Autodesk Inventor part; units mm, degrees
(part 3 of 5)
  spline S419 degree 2 poles (-346.7745, 60.714) (-347.3687, 60.714) (-348.0307, 61.3279) (-348.0307, 61.8712) knots 0 0 0 1 2 2 2
  spline S420 degree 2 poles (-348.0307, 61.8712) (-348.0307, 62.2163) (-347.7195, 62.7284) (-347.1452, 63) (-346.7717, 63) knots 0 0 0 1 2 3 3 3
  spline S421 degree 2 poles (-346.7717, 63) (-346.3841, 63) (-345.8154, 62.7143) (-345.5126, 62.2078) (-345.5126, 61.8966) knots 0 0 0 1 2 3 3 3
  spline S422 degree 2 poles (-346.4322, 61.891) (-346.4322, 62.3352) (-346.7717, 62.3352) knots 0 0 0 1 1 1
  spline S423 degree 2 poles (-346.7717, 62.3352) (-347.1112, 62.3352) (-347.1112, 61.8712) knots 0 0 0 1 1 1
  spline S424 degree 2 poles (-347.1112, 61.8712) (-347.1112, 61.3789) (-346.766, 61.3789) knots 0 0 0 1 1 1
  spline S425 degree 2 poles (-346.766, 61.3789) (-346.4322, 61.3789) (-346.4322, 61.891) knots 0 0 0 1 1 1
  spline S426 degree 2 poles (-398.07, 55.8694) (-398.07, 55.7053) (-398.2397, 55.4139) (-398.5311, 55.247) (-398.6924, 55.247) knots 0 0 0 1 2 3 3 3
  spline S427 degree 2 poles (-398.6924, 55.247) (-398.9442, 55.247) (-399.3064, 55.6091) (-399.3064, 55.8694) knots 0 0 0 1 2 2 2
  spline S428 degree 2 poles (-399.3064, 55.8694) (-399.3064, 56.1212) (-398.9499, 56.4834) (-398.6924, 56.4834) knots 0 0 0 1 2 2 2
  spline S429 degree 2 poles (-398.6924, 56.4834) (-398.4293, 56.4834) (-398.07, 56.1156) (-398.07, 55.8694) knots 0 0 0 1 2 2 2
  spline S430 degree 2 poles (-387.3157, 56.3957) (-387.3157, 55.9317) (-387.7062, 55.2187) (-388.4277, 54.8311) (-388.9002, 54.8311) knots 0 0 0 1 2 3 3 3
  line L463 (-388.9002, 54.8311) -> (-390.1932, 54.8311)
  line L464 (-390.1932, 54.8311) -> (-390.1932, 57.8811)
  line L465 (-390.1932, 57.8811) -> (-388.9285, 57.8811)
  spline S431 degree 2 poles (-388.9285, 57.8811) (-387.3157, 57.8811) (-387.3157, 56.3957) knots 0 0 0 1 1 1
  spline S432 degree 2 poles (-388.2919, 56.3872) (-388.2919, 56.6079) (-388.4729, 56.9672) (-388.8096, 57.1624) (-389.036, 57.1624) knots 0 0 0 1 2 3 3 3
  line L466 (-389.036, 57.1624) -> (-389.2736, 57.1624)
  line L467 (-389.2736, 57.1624) -> (-389.2736, 55.5497)
  line L468 (-389.2736, 55.5497) -> (-389.0162, 55.5497)
  spline S433 degree 2 poles (-389.0162, 55.5497) (-388.6851, 55.5497) (-388.2919, 56.0024) (-388.2919, 56.3872) knots 0 0 0 1 2 2 2
  spline S434 degree 2 poles (-386.1868, 55.6629) (-386.1642, 55.5214) (-385.8869, 55.363) (-385.6606, 55.363) knots 0 0 0 1 2 2 2
  spline S435 degree 2 poles (-385.6606, 55.363) (-385.3437, 55.363) (-385.0608, 55.4846) knots 0 0 0 1 1 1
  line L469 (-385.0608, 55.4846) -> (-385.0608, 54.9103)
  spline S436 degree 2 poles (-385.0608, 54.9103) (-385.389, 54.7773) (-385.8615, 54.7773) knots 0 0 0 1 1 1
  spline S437 degree 2 poles (-385.8615, 54.7773) (-386.4302, 54.7773) (-387.0639, 55.3601) (-387.0639, 55.8722) knots 0 0 0 1 2 2 2
  spline S438 degree 2 poles (-387.0639, 55.8722) (-387.0639, 56.2231) (-386.7867, 56.7578) (-386.2406, 57.0634) (-385.9096, 57.0634) knots 0 0 0 1 2 3 3 3
  spline S439 degree 2 poles (-385.9096, 57.0634) (-385.5729, 57.0634) (-385.0919, 56.8003) (-384.8429, 56.3221) (-384.8429, 56.0024) knots 0 0 0 1 2 3 3 3
  line L470 (-384.8429, 56.0024) -> (-384.8429, 55.6629)
  line L471 (-384.8429, 55.6629) -> (-386.1868, 55.6629)
  spline S440 degree 2 poles (-385.6436, 56.1382) (-385.6436, 56.5145) (-385.9124, 56.5145) knots 0 0 0 1 1 1
  spline S441 degree 2 poles (-385.9124, 56.5145) (-386.0256, 56.5145) (-386.1784, 56.308) (-386.1925, 56.1382) knots 0 0 0 1 2 2 2
  line L472 (-386.1925, 56.1382) -> (-385.6436, 56.1382)
  line L473 (-384.5289, 54.8311) -> (-384.5289, 58.0565)
  line L474 (-384.5289, 58.0565) -> (-383.6235, 58.0565)
  line L475 (-383.6235, 58.0565) -> (-383.6235, 54.8311)
  line L476 (-383.6235, 54.8311) -> (-384.5289, 54.8311)
  spline S442 degree 2 poles (-379.3993, 56.8766) (-379.3993, 56.5626) (-379.7162, 56.0788) (-380.3047, 55.8128) (-380.6952, 55.8128) knots 0 0 0 1 2 3 3 3
  line L477 (-380.6952, 55.8128) -> (-380.9753, 55.8128)
  line L478 (-380.9753, 55.8128) -> (-380.9753, 54.8311)
  line L479 (-380.9753, 54.8311) -> (-381.8948, 54.8311)
  line L480 (-381.8948, 54.8311) -> (-381.8948, 57.8811)
  line L481 (-381.8948, 57.8811) -> (-380.6414, 57.8811)
  spline S443 degree 2 poles (-380.6414, 57.8811) (-379.9963, 57.8811) (-379.3993, 57.3916) (-379.3993, 56.8766) knots 0 0 0 1 2 2 2
  spline S444 degree 2 poles (-380.3726, 56.8427) (-380.3726, 57.0294) (-380.5905, 57.2218) (-380.7998, 57.2218) knots 0 0 0 1 2 2 2
  line L482 (-380.7998, 57.2218) -> (-380.9753, 57.2218)
  line L483 (-380.9753, 57.2218) -> (-380.9753, 56.4692)
  line L484 (-380.9753, 56.4692) -> (-380.7687, 56.4692)
  spline S445 degree 2 poles (-380.7687, 56.4692) (-380.3726, 56.4692) (-380.3726, 56.8427) knots 0 0 0 1 1 1
  line L485 (-377.9111, 54.8311) -> (-377.9111, 55.1621)
  line L486 (-377.9111, 55.1621) -> (-377.9196, 55.1621)
  spline S446 degree 2 poles (-377.9196, 55.1621) (-378.1375, 54.7773) (-378.5845, 54.7773) knots 0 0 0 1 1 1
  spline S447 degree 2 poles (-378.5845, 54.7773) (-378.8929, 54.7773) (-379.2409, 55.1423) (-379.2409, 55.4507) knots 0 0 0 1 2 2 2
  spline S448 degree 2 poles (-379.2409, 55.4507) (-379.2409, 56.0929) (-378.4515, 56.1948) knots 0 0 0 1 1 1
  line L487 (-378.4515, 56.1948) -> (-377.9111, 56.2655)
  spline S449 degree 2 poles (-377.9111, 56.2655) (-377.9111, 56.373) (-378.1035, 56.5088) (-378.2648, 56.5088) knots 0 0 0 1 2 2 2
  spline S450 degree 2 poles (-378.2648, 56.5088) (-378.6298, 56.5088) (-379.0372, 56.2995) knots 0 0 0 1 1 1
  line L488 (-379.0372, 56.2995) -> (-379.0372, 56.888)
  spline S451 degree 2 poles (-379.0372, 56.888) (-378.8618, 56.9644) (-378.327, 57.0634) (-378.1375, 57.0634) knots 0 0 0 1 2 2 2
  spline S452 degree 2 poles (-378.1375, 57.0634) (-377.5829, 57.0634) (-377.0821, 56.5881) (-377.0821, 56.0335) knots 0 0 0 1 2 2 2
  line L489 (-377.0821, 56.0335) -> (-377.0821, 54.8311)
  line L490 (-377.0821, 54.8311) -> (-377.9111, 54.8311)
  spline S453 degree 2 poles (-378.4487, 55.5723) (-378.4487, 55.4846) (-378.3355, 55.3686) (-378.2308, 55.3686) knots 0 0 0 1 2 2 2
  spline S454 degree 2 poles (-378.2308, 55.3686) (-378.0894, 55.3686) (-377.9111, 55.5808) (-377.9111, 55.7478) knots 0 0 0 1 2 2 2
  line L491 (-377.9111, 55.7478) -> (-377.9111, 55.8298)
  line L492 (-377.9111, 55.8298) -> (-378.2195, 55.7874)
  spline S455 degree 2 poles (-378.2195, 55.7874) (-378.4487, 55.7478) (-378.4487, 55.5723) knots 0 0 0 1 1 1
  spline S456 degree 2 poles (-374.2189, 55.9854) (-374.2189, 55.6289) (-374.4622, 55.08) (-374.9035, 54.7773) (-375.1808, 54.7773) knots 0 0 0 1 2 3 3 3
  spline S457 degree 2 poles (-375.1808, 54.7773) (-375.5628, 54.7773) (-375.7608, 55.0574) knots 0 0 0 1 1 1
  line L493 (-375.7608, 55.0574) -> (-375.7693, 55.0574)
  line L494 (-375.7693, 55.0574) -> (-375.7693, 53.8295)
  line L495 (-375.7693, 53.8295) -> (-376.6747, 53.8295)
  line L496 (-376.6747, 53.8295) -> (-376.6747, 57.0096)
  line L497 (-376.6747, 57.0096) -> (-375.7693, 57.0096)
  line L498 (-375.7693, 57.0096) -> (-375.7693, 56.7125)
  line L499 (-375.7693, 56.7125) -> (-375.7608, 56.7125)
  spline S458 degree 2 poles (-375.7608, 56.7125) (-375.6533, 56.8766) (-375.3081, 57.0634) (-375.0875, 57.0634) knots 0 0 0 1 2 2 2
  spline S459 degree 2 poles (-375.0875, 57.0634) (-374.6687, 57.0634) (-374.2189, 56.5004) (-374.2189, 55.9854) knots 0 0 0 1 2 2 2
  spline S460 degree 2 poles (-375.1384, 55.96) (-375.1384, 56.1637) (-375.2968, 56.3985) (-375.4638, 56.3985) knots 0 0 0 1 2 2 2
  spline S461 degree 2 poles (-375.4638, 56.3985) (-375.608, 56.3985) (-375.7863, 56.1523) (-375.7863, 55.9373) knots 0 0 0 1 2 2 2
  line L500 (-375.7863, 55.9373) -> (-375.7863, 55.8949)
  spline S462 degree 2 poles (-375.7863, 55.8949) (-375.7863, 55.6883) (-375.6335, 55.4422) (-375.4807, 55.4422) knots 0 0 0 1 2 2 2
  spline S463 degree 2 poles (-375.4807, 55.4422) (-375.3166, 55.4422) (-375.1384, 55.711) (-375.1384, 55.96) knots 0 0 0 1 2 2 2
  line L501 (-372.6684, 54.8311) -> (-372.6684, 55.1621)
  line L502 (-372.6684, 55.1621) -> (-372.6769, 55.1621)
  spline S464 degree 2 poles (-372.6769, 55.1621) (-372.8947, 54.7773) (-373.3418, 54.7773) knots 0 0 0 1 1 1
  spline S465 degree 2 poles (-373.3418, 54.7773) (-373.6502, 54.7773) (-373.9982, 55.1423) (-373.9982, 55.4507) knots 0 0 0 1 2 2 2
  spline S466 degree 2 poles (-373.9982, 55.4507) (-373.9982, 56.0929) (-373.2088, 56.1948) knots 0 0 0 1 1 1
  line L503 (-373.2088, 56.1948) -> (-372.6684, 56.2655)
  spline S467 degree 2 poles (-372.6684, 56.2655) (-372.6684, 56.373) (-372.8608, 56.5088) (-373.0221, 56.5088) knots 0 0 0 1 2 2 2
  spline S468 degree 2 poles (-373.0221, 56.5088) (-373.387, 56.5088) (-373.7945, 56.2995) knots 0 0 0 1 1 1
  line L504 (-373.7945, 56.2995) -> (-373.7945, 56.888)
  spline S469 degree 2 poles (-373.7945, 56.888) (-373.619, 56.9644) (-373.0843, 57.0634) (-372.8947, 57.0634) knots 0 0 0 1 2 2 2
  spline S470 degree 2 poles (-372.8947, 57.0634) (-372.3402, 57.0634) (-371.8394, 56.5881) (-371.8394, 56.0335) knots 0 0 0 1 2 2 2
  line L505 (-371.8394, 56.0335) -> (-371.8394, 54.8311)
  line L506 (-371.8394, 54.8311) -> (-372.6684, 54.8311)
  line L507 (-373.0277, 57.3548) -> (-373.786, 58.0367)
  line L508 (-373.786, 58.0367) -> (-373.0249, 58.0367)
  line L509 (-373.0249, 58.0367) -> (-372.3883, 57.3548)
  line L510 (-372.3883, 57.3548) -> (-373.0277, 57.3548)
  spline S471 degree 2 poles (-373.206, 55.5723) (-373.206, 55.4846) (-373.0928, 55.3686) (-372.9881, 55.3686) knots 0 0 0 1 2 2 2
  spline S472 degree 2 poles (-372.9881, 55.3686) (-372.8466, 55.3686) (-372.6684, 55.5808) (-372.6684, 55.7478) knots 0 0 0 1 2 2 2
  line L511 (-372.6684, 55.7478) -> (-372.6684, 55.8298)
  line L512 (-372.6684, 55.8298) -> (-372.9768, 55.7874)
  spline S473 degree 2 poles (-372.9768, 55.7874) (-373.206, 55.7478) (-373.206, 55.5723) knots 0 0 0 1 1 1
  line L513 (-368.0085, 54.8311) -> (-369.0836, 56.3023)
  spline S474 degree 2 poles (-369.0836, 56.3023) (-369.211, 56.4749) (-369.293, 56.6164) knots 0 0 0 1 1 1
  line L514 (-369.293, 56.6164) -> (-369.3015, 56.6164)
  spline S475 degree 2 poles (-369.3015, 56.6164) (-369.2874, 56.39) (-369.2874, 56.1099) knots 0 0 0 1 1 1
  line L515 (-369.2874, 56.1099) -> (-369.2874, 54.8311)
  line L516 (-369.2874, 54.8311) -> (-370.139, 54.8311)
  line L517 (-370.139, 54.8311) -> (-370.139, 57.8811)
  line L518 (-370.139, 57.8811) -> (-369.2704, 57.8811)
  line L519 (-369.2704, 57.8811) -> (-368.2405, 56.4805)
  spline S476 degree 2 poles (-368.2405, 56.4805) (-368.2207, 56.4523) (-368.1641, 56.3759) (-368.1104, 56.2966) (-368.0623, 56.2202) (-368.0481, 56.1891) knots 0 0 0 1 2 3 4 4 4
  line L520 (-368.0481, 56.1891) -> (-368.0396, 56.1891)
  spline S477 degree 2 poles (-368.0396, 56.1891) (-368.0538, 56.2825) (-368.0538, 56.5117) knots 0 0 0 1 1 1
  line L521 (-368.0538, 56.5117) -> (-368.0538, 57.8811)
  line L522 (-368.0538, 57.8811) -> (-367.2022, 57.8811)
  line L523 (-367.2022, 57.8811) -> (-367.2022, 54.8311)
  line L524 (-367.2022, 54.8311) -> (-368.0085, 54.8311)
  line L525 (-366.6844, 54.8311) -> (-366.6844, 57.0096)
  line L526 (-366.6844, 57.0096) -> (-365.779, 57.0096)
  line L527 (-365.779, 57.0096) -> (-365.779, 54.8311)
  line L528 (-365.779, 54.8311) -> (-366.6844, 54.8311)
  spline S478 degree 2 poles (-365.7253, 57.5981) (-365.7253, 57.4057) (-366.0054, 57.1681) (-366.2317, 57.1681) knots 0 0 0 1 2 2 2
  spline S479 degree 2 poles (-366.2317, 57.1681) (-366.4524, 57.1681) (-366.7353, 57.4142) (-366.7353, 57.5981) knots 0 0 0 1 2 2 2
  spline S480 degree 2 poles (-366.7353, 57.5981) (-366.7353, 57.7849) (-366.4609, 58.0169) (-366.2317, 58.0169) knots 0 0 0 1 2 2 2
  spline S481 degree 2 poles (-366.2317, 58.0169) (-366.0054, 58.0169) (-365.7253, 57.7849) (-365.7253, 57.5981) knots 0 0 0 1 2 2 2
  spline S482 degree 2 poles (-363.5495, 54.8933) (-363.6372, 54.8424) (-364.0107, 54.7773) (-364.254, 54.7773) knots 0 0 0 1 2 2 2
  spline S483 degree 2 poles (-364.254, 54.7773) (-364.5992, 54.7773) (-365.1424, 55.0574) (-365.4395, 55.5582) (-365.4395, 55.8722) knots 0 0 0 1 2 3 3 3
  spline S484 degree 2 poles (-365.4395, 55.8722) (-365.4395, 56.2457) (-365.1226, 56.7805) (-364.5369, 57.0634) (-364.1493, 57.0634) knots 0 0 0 1 2 3 3 3
  spline S485 degree 2 poles (-364.1493, 57.0634) (-363.9371, 57.0634) (-363.5976, 57.0068) (-363.5495, 56.9728) knots 0 0 0 1 2 2 2
  line L529 (-363.5495, 56.9728) -> (-363.5495, 56.2655)
  spline S486 degree 2 poles (-363.5495, 56.2655) (-363.6174, 56.3193) (-363.8721, 56.3985) (-363.9796, 56.3985) knots 0 0 0 1 2 2 2
  spline S487 degree 2 poles (-363.9796, 56.3985) (-364.2455, 56.3985) (-364.52, 56.1467) (-364.52, 55.9175) knots 0 0 0 1 2 2 2
  spline S488 degree 2 poles (-364.52, 55.9175) (-364.52, 55.6912) (-364.2512, 55.4422) (-364.0135, 55.4422) knots 0 0 0 1 2 2 2
  spline S489 degree 2 poles (-364.0135, 55.4422) (-363.7617, 55.4422) (-363.5495, 55.561) knots 0 0 0 1 1 1
  line L530 (-363.5495, 55.561) -> (-363.5495, 54.8933)
  spline S490 degree 2 poles (-360.7655, 55.96) (-360.7655, 55.4082) (-361.4304, 54.7773) (-362.0273, 54.7773) knots 0 0 0 1 2 2 2
  spline S491 degree 2 poles (-362.0273, 54.7773) (-362.6215, 54.7773) (-363.2836, 55.3913) (-363.2836, 55.9345) knots 0 0 0 1 2 2 2
  spline S492 degree 2 poles (-363.2836, 55.9345) (-363.2836, 56.2797) (-362.9723, 56.7918) (-362.398, 57.0634) (-362.0245, 57.0634) knots 0 0 0 1 2 3 3 3
  spline S493 degree 2 poles (-362.0245, 57.0634) (-361.6369, 57.0634) (-361.0682, 56.7776) (-360.7655, 56.2712) (-360.7655, 55.96) knots 0 0 0 1 2 3 3 3
  spline S494 degree 2 poles (-361.685, 55.9543) (-361.685, 56.3985) (-362.0245, 56.3985) knots 0 0 0 1 1 1
  spline S495 degree 2 poles (-362.0245, 56.3985) (-362.364, 56.3985) (-362.364, 55.9345) knots 0 0 0 1 1 1
  spline S496 degree 2 poles (-362.364, 55.9345) (-362.364, 55.4422) (-362.0189, 55.4422) knots 0 0 0 1 1 1
  spline S497 degree 2 poles (-362.0189, 55.4422) (-361.685, 55.4422) (-361.685, 55.9543) knots 0 0 0 1 1 1
  line L531 (-360.4259, 54.8311) -> (-360.4259, 58.0565)
  line L532 (-360.4259, 58.0565) -> (-359.5206, 58.0565)
  line L533 (-359.5206, 58.0565) -> (-359.5206, 54.8311)
  line L534 (-359.5206, 54.8311) -> (-360.4259, 54.8311)
  spline S498 degree 2 poles (-356.663, 55.96) (-356.663, 55.4082) (-357.3279, 54.7773) (-357.9248, 54.7773) knots 0 0 0 1 2 2 2
  spline S499 degree 2 poles (-357.9248, 54.7773) (-358.519, 54.7773) (-359.1811, 55.3913) (-359.1811, 55.9345) knots 0 0 0 1 2 2 2
  spline S500 degree 2 poles (-359.1811, 55.9345) (-359.1811, 56.2797) (-358.8698, 56.7918) (-358.2955, 57.0634) (-357.922, 57.0634) knots 0 0 0 1 2 3 3 3
  spline S501 degree 2 poles (-357.922, 57.0634) (-357.5344, 57.0634) (-356.9657, 56.7776) (-356.663, 56.2712) (-356.663, 55.96) knots 0 0 0 1 2 3 3 3
  spline S502 degree 2 poles (-357.5825, 55.9543) (-357.5825, 56.3985) (-357.922, 56.3985) knots 0 0 0 1 1 1
  spline S503 degree 2 poles (-357.922, 56.3985) (-358.2615, 56.3985) (-358.2615, 55.9345) knots 0 0 0 1 1 1
  spline S504 degree 2 poles (-358.2615, 55.9345) (-358.2615, 55.4422) (-357.9163, 55.4422) knots 0 0 0 1 1 1
  spline S505 degree 2 poles (-357.9163, 55.4422) (-357.5825, 55.4422) (-357.5825, 55.9543) knots 0 0 0 1 1 1
  line L535 (-358.0295, 57.3548) -> (-358.7878, 58.0367)
  line L536 (-358.7878, 58.0367) -> (-358.0267, 58.0367)
  line L537 (-358.0267, 58.0367) -> (-357.3901, 57.3548)
  line L538 (-357.3901, 57.3548) -> (-358.0295, 57.3548)
  spline S506 degree 2 poles (-398.07, 49.9327) (-398.07, 49.7686) (-398.2397, 49.4772) (-398.5311, 49.3103) (-398.6924, 49.3103) knots 0 0 0 1 2 3 3 3
  spline S507 degree 2 poles (-398.6924, 49.3103) (-398.9442, 49.3103) (-399.3064, 49.6725) (-399.3064, 49.9327) knots 0 0 0 1 2 2 2
  spline S508 degree 2 poles (-399.3064, 49.9327) (-399.3064, 50.1846) (-398.9499, 50.5467) (-398.6924, 50.5467) knots 0 0 0 1 2 2 2
  spline S509 degree 2 poles (-398.6924, 50.5467) (-398.4293, 50.5467) (-398.07, 50.1789) (-398.07, 49.9327) knots 0 0 0 1 2 2 2
  spline S510 degree 2 poles (-387.3157, 50.459) (-387.3157, 49.995) (-387.7062, 49.282) (-388.4277, 48.8944) (-388.9002, 48.8944) knots 0 0 0 1 2 3 3 3
  line L539 (-388.9002, 48.8944) -> (-390.1932, 48.8944)
  line L540 (-390.1932, 48.8944) -> (-390.1932, 51.9444)
  line L541 (-390.1932, 51.9444) -> (-388.9285, 51.9444)
  spline S511 degree 2 poles (-388.9285, 51.9444) (-387.3157, 51.9444) (-387.3157, 50.459) knots 0 0 0 1 1 1
  spline S512 degree 2 poles (-388.2919, 50.4505) (-388.2919, 50.6712) (-388.4729, 51.0305) (-388.8096, 51.2257) (-389.036, 51.2257) knots 0 0 0 1 2 3 3 3
  line L542 (-389.036, 51.2257) -> (-389.2736, 51.2257)
  line L543 (-389.2736, 51.2257) -> (-389.2736, 49.613)
  line L544 (-389.2736, 49.613) -> (-389.0162, 49.613)
  spline S513 degree 2 poles (-389.0162, 49.613) (-388.6851, 49.613) (-388.2919, 50.0657) (-388.2919, 50.4505) knots 0 0 0 1 2 2 2
  line L545 (-386.9677, 48.8944) -> (-386.9677, 51.073)
  line L546 (-386.9677, 51.073) -> (-386.0624, 51.073)
  line L547 (-386.0624, 51.073) -> (-386.0624, 48.8944)
  line L548 (-386.0624, 48.8944) -> (-386.9677, 48.8944)
  spline S514 degree 2 poles (-386.0086, 51.6615) (-386.0086, 51.4691) (-386.2887, 51.2314) (-386.515, 51.2314) knots 0 0 0 1 2 2 2
  spline S515 degree 2 poles (-386.515, 51.2314) (-386.7357, 51.2314) (-387.0187, 51.4776) (-387.0187, 51.6615) knots 0 0 0 1 2 2 2
  spline S516 degree 2 poles (-387.0187, 51.6615) (-387.0187, 51.8482) (-386.7442, 52.0802) (-386.515, 52.0802) knots 0 0 0 1 2 2 2
  spline S517 degree 2 poles (-386.515, 52.0802) (-386.2887, 52.0802) (-386.0086, 51.8482) (-386.0086, 51.6615) knots 0 0 0 1 2 2 2
  line L549 (-382.5936, 48.8944) -> (-383.6263, 48.8944)
  line L550 (-383.6263, 48.8944) -> (-384.6109, 51.9444)
  line L551 (-384.6109, 51.9444) -> (-383.6235, 51.9444)
  line L552 (-383.6235, 51.9444) -> (-383.1567, 50.0657)
  spline S518 degree 2 poles (-383.1567, 50.0657) (-383.1001, 49.8394) (-383.0944, 49.7262) knots 0 0 0 1 1 1
  line L553 (-383.0944, 49.7262) -> (-383.0746, 49.7262)
  spline S519 degree 2 poles (-383.0746, 49.7262) (-383.0605, 49.8677) (-383.0067, 50.0799) knots 0 0 0 1 1 1
  line L554 (-383.0067, 50.0799) -> (-382.554, 51.9444)
  line L555 (-382.554, 51.9444) -> (-381.5977, 51.9444)
  line L556 (-381.5977, 51.9444) -> (-382.5936, 48.8944)
  line L557 (-381.3572, 48.8944) -> (-381.3572, 51.073)
  line L558 (-381.3572, 51.073) -> (-380.4518, 51.073)
  line L559 (-380.4518, 51.073) -> (-380.4518, 48.8944)
  line L560 (-380.4518, 48.8944) -> (-381.3572, 48.8944)
  spline S520 degree 2 poles (-380.3981, 51.6615) (-380.3981, 51.4691) (-380.6782, 51.2314) (-380.9045, 51.2314) knots 0 0 0 1 2 2 2
  spline S521 degree 2 poles (-380.9045, 51.2314) (-381.1252, 51.2314) (-381.4081, 51.4776) (-381.4081, 51.6615) knots 0 0 0 1 2 2 2
  spline S522 degree 2 poles (-381.4081, 51.6615) (-381.4081, 51.8482) (-381.1337, 52.0802) (-380.9045, 52.0802) knots 0 0 0 1 2 2 2
  spline S523 degree 2 poles (-380.9045, 52.0802) (-380.6782, 52.0802) (-380.3981, 51.8482) (-380.3981, 51.6615) knots 0 0 0 1 2 2 2
  line L561 (-378.6043, 48.8944) -> (-378.6043, 50.0827)
  spline S524 degree 2 poles (-378.6043, 50.0827) (-378.6043, 50.2864) (-378.7259, 50.4618) (-378.8618, 50.4618) knots 0 0 0 1 2 2 2
  spline S525 degree 2 poles (-378.8618, 50.4618) (-378.9778, 50.4618) (-379.1107, 50.2779) (-379.1107, 50.1365) knots 0 0 0 1 2 2 2
  line L562 (-379.1107, 50.1365) -> (-379.1107, 48.8944)
  line L563 (-379.1107, 48.8944) -> (-380.0161, 48.8944)
  line L564 (-380.0161, 48.8944) -> (-380.0161, 51.073)
  line L565 (-380.0161, 51.073) -> (-379.1107, 51.073)
  line L566 (-379.1107, 51.073) -> (-379.1107, 50.7334)
  line L567 (-379.1107, 50.7334) -> (-379.1022, 50.7334)
  spline S526 degree 2 poles (-379.1022, 50.7334) (-378.9947, 50.9202) (-378.6269, 51.1267) (-378.4119, 51.1267) knots 0 0 0 1 2 2 2
  spline S527 degree 2 poles (-378.4119, 51.1267) (-377.6989, 51.1267) (-377.6989, 50.2242) knots 0 0 0 1 1 1
  line L568 (-377.6989, 50.2242) -> (-377.6989, 48.8944)
  line L569 (-377.6989, 48.8944) -> (-378.6043, 48.8944)
  spline S528 degree 2 poles (-375.4949, 48.9566) (-375.5826, 48.9057) (-375.9561, 48.8406) (-376.1994, 48.8406) knots 0 0 0 1 2 2 2
  spline S529 degree 2 poles (-376.1994, 48.8406) (-376.5445, 48.8406) (-377.0878, 49.1207) (-377.3849, 49.6215) (-377.3849, 49.9356) knots 0 0 0 1 2 3 3 3
  spline S530 degree 2 poles (-377.3849, 49.9356) (-377.3849, 50.309) (-377.068, 50.8438) (-376.4823, 51.1267) (-376.0947, 51.1267) knots 0 0 0 1 2 3 3 3
  spline S531 degree 2 poles (-376.0947, 51.1267) (-375.8825, 51.1267) (-375.543, 51.0701) (-375.4949, 51.0362) knots 0 0 0 1 2 2 2
  line L570 (-375.4949, 51.0362) -> (-375.4949, 50.3289)
  spline S532 degree 2 poles (-375.4949, 50.3289) (-375.5628, 50.3826) (-375.8174, 50.4618) (-375.9249, 50.4618) knots 0 0 0 1 2 2 2
  spline S533 degree 2 poles (-375.9249, 50.4618) (-376.1909, 50.4618) (-376.4653, 50.21) (-376.4653, 49.9808) knots 0 0 0 1 2 2 2
  spline S534 degree 2 poles (-376.4653, 49.9808) (-376.4653, 49.7545) (-376.1965, 49.5055) (-375.9589, 49.5055) knots 0 0 0 1 2 2 2
  spline S535 degree 2 poles (-375.9589, 49.5055) (-375.7071, 49.5055) (-375.4949, 49.6244) knots 0 0 0 1 1 1
  line L571 (-375.4949, 49.6244) -> (-375.4949, 48.9566)
  spline S536 degree 2 poles (-374.3518, 49.7262) (-374.3292, 49.5847) (-374.0519, 49.4263) (-373.8256, 49.4263) knots 0 0 0 1 2 2 2
  spline S537 degree 2 poles (-373.8256, 49.4263) (-373.5087, 49.4263) (-373.2258, 49.548) knots 0 0 0 1 1 1
  line L572 (-373.2258, 49.548) -> (-373.2258, 48.9736)
  spline S538 degree 2 poles (-373.2258, 48.9736) (-373.554, 48.8406) (-374.0265, 48.8406) knots 0 0 0 1 1 1
  spline S539 degree 2 poles (-374.0265, 48.8406) (-374.5952, 48.8406) (-375.2289, 49.4235) (-375.2289, 49.9356) knots 0 0 0 1 2 2 2
  spline S540 degree 2 poles (-375.2289, 49.9356) (-375.2289, 50.2864) (-374.9516, 50.8212) (-374.4056, 51.1267) (-374.0746, 51.1267) knots 0 0 0 1 2 3 3 3
  spline S541 degree 2 poles (-374.0746, 51.1267) (-373.7379, 51.1267) (-373.2569, 50.8636) (-373.0079, 50.3854) (-373.0079, 50.0657) knots 0 0 0 1 2 3 3 3
  line L573 (-373.0079, 50.0657) -> (-373.0079, 49.7262)
  line L574 (-373.0079, 49.7262) -> (-374.3518, 49.7262)
  spline S542 degree 2 poles (-373.8086, 50.2015) (-373.8086, 50.5778) (-374.0774, 50.5778) knots 0 0 0 1 1 1
  spline S543 degree 2 poles (-374.0774, 50.5778) (-374.1906, 50.5778) (-374.3433, 50.3713) (-374.3575, 50.2015) knots 0 0 0 1 2 2 2
  line L575 (-374.3575, 50.2015) -> (-373.8086, 50.2015)
  line L576 (-371.282, 48.8944) -> (-371.282, 50.0827)
  spline S544 degree 2 poles (-371.282, 50.0827) (-371.282, 50.2864) (-371.4037, 50.4618) (-371.5395, 50.4618) knots 0 0 0 1 2 2 2
  spline S545 degree 2 poles (-371.5395, 50.4618) (-371.6555, 50.4618) (-371.7885, 50.2779) (-371.7885, 50.1365) knots 0 0 0 1 2 2 2
  line L577 (-371.7885, 50.1365) -> (-371.7885, 48.8944)
  line L578 (-371.7885, 48.8944) -> (-372.6939, 48.8944)
  line L579 (-372.6939, 48.8944) -> (-372.6939, 51.073)
  line L580 (-372.6939, 51.073) -> (-371.7885, 51.073)
  line L581 (-371.7885, 51.073) -> (-371.7885, 50.7334)
  line L582 (-371.7885, 50.7334) -> (-371.78, 50.7334)
  spline S546 degree 2 poles (-371.78, 50.7334) (-371.6725, 50.9202) (-371.3047, 51.1267) (-371.0896, 51.1267) knots 0 0 0 1 2 2 2
  spline S547 degree 2 poles (-371.0896, 51.1267) (-370.3766, 51.1267) (-370.3766, 50.2242) knots 0 0 0 1 1 1
  line L583 (-370.3766, 50.2242) -> (-370.3766, 48.8944)
  line L584 (-370.3766, 48.8944) -> (-371.282, 48.8944)
  line L585 (-368.9422, 49.5225) -> (-368.0453, 49.5225)
  line L586 (-368.0453, 49.5225) -> (-368.0453, 48.8944)
  line L587 (-368.0453, 48.8944) -> (-370.1305, 48.8944)
  line L588 (-370.1305, 48.8944) -> (-370.1305, 49.3131)
  line L589 (-370.1305, 49.3131) -> (-369.1516, 50.4449)
  line L590 (-369.1516, 50.4449) -> (-370.04, 50.4449)
  line L591 (-370.04, 50.4449) -> (-370.04, 51.073)
  line L592 (-370.04, 51.073) -> (-368.0651, 51.073)
  line L593 (-368.0651, 51.073) -> (-368.0651, 50.558)
  line L594 (-368.0651, 50.558) -> (-368.9422, 49.5225)
  spline S548 degree 2 poles (-365.3263, 50.0233) (-365.3263, 49.4716) (-365.9912, 48.8406) (-366.5882, 48.8406) knots 0 0 0 1 2 2 2
  spline S549 degree 2 poles (-366.5882, 48.8406) (-367.1823, 48.8406) (-367.8444, 49.4546) (-367.8444, 49.9978) knots 0 0 0 1 2 2 2
  spline S550 degree 2 poles (-367.8444, 49.9978) (-367.8444, 50.343) (-367.5332, 50.8551) (-366.9588, 51.1267) (-366.5854, 51.1267) knots 0 0 0 1 2 3 3 3
  spline S551 degree 2 poles (-366.5854, 51.1267) (-366.1977, 51.1267) (-365.6291, 50.841) (-365.3263, 50.3345) (-365.3263, 50.0233) knots 0 0 0 1 2 3 3 3
  spline S552 degree 2 poles (-366.2458, 50.0176) (-366.2458, 50.4618) (-366.5854, 50.4618) knots 0 0 0 1 1 1
  spline S553 degree 2 poles (-366.5854, 50.4618) (-366.9249, 50.4618) (-366.9249, 49.9978) knots 0 0 0 1 1 1
  spline S554 degree 2 poles (-366.9249, 49.9978) (-366.9249, 49.5055) (-366.5797, 49.5055) knots 0 0 0 1 1 1
  spline S555 degree 2 poles (-366.5797, 49.5055) (-366.2458, 49.5055) (-366.2458, 50.0176) knots 0 0 0 1 1 1
  line L595 (-362.7743, 51.2257) -> (-362.7743, 50.6769)
  line L596 (-362.7743, 50.6769) -> (-361.8689, 50.6769)
  line L597 (-361.8689, 50.6769) -> (-361.8689, 49.9582)
  line L598 (-361.8689, 49.9582) -> (-362.7743, 49.9582)
  line L599 (-362.7743, 49.9582) -> (-362.7743, 48.8944)
  line L600 (-362.7743, 48.8944) -> (-363.6938, 48.8944)
  line L601 (-363.6938, 48.8944) -> (-363.6938, 51.9444)
  line L602 (-363.6938, 51.9444) -> (-361.7812, 51.9444)
  line L603 (-361.7812, 51.9444) -> (-361.7812, 51.2257)
  line L604 (-361.7812, 51.2257) -> (-362.7743, 51.2257)
  line L605 (-360.2109, 48.8944) -> (-360.2109, 49.2254)
  line L606 (-360.2109, 49.2254) -> (-360.2194, 49.2254)
  spline S556 degree 2 poles (-360.2194, 49.2254) (-360.4373, 48.8406) (-360.8843, 48.8406) knots 0 0 0 1 1 1
  spline S557 degree 2 poles (-360.8843, 48.8406) (-361.1927, 48.8406) (-361.5407, 49.2056) (-361.5407, 49.514) knots 0 0 0 1 2 2 2
  spline S558 degree 2 poles (-361.5407, 49.514) (-361.5407, 50.1563) (-360.7513, 50.2581) knots 0 0 0 1 1 1
  line L607 (-360.7513, 50.2581) -> (-360.2109, 50.3289)
  spline S559 degree 2 poles (-360.2109, 50.3289) (-360.2109, 50.4364) (-360.4033, 50.5722) (-360.5646, 50.5722) knots 0 0 0 1 2 2 2
  spline S560 degree 2 poles (-360.5646, 50.5722) (-360.9296, 50.5722) (-361.337, 50.3628) knots 0 0 0 1 1 1
  line L608 (-361.337, 50.3628) -> (-361.337, 50.9513)
  spline S561 degree 2 poles (-361.337, 50.9513) (-361.1616, 51.0277) (-360.6268, 51.1267) (-360.4373, 51.1267) knots 0 0 0 1 2 2 2
  spline S562 degree 2 poles (-360.4373, 51.1267) (-359.8827, 51.1267) (-359.3819, 50.6514) (-359.3819, 50.0968) knots 0 0 0 1 2 2 2
  line L609 (-359.3819, 50.0968) -> (-359.3819, 48.8944)
  line L610 (-359.3819, 48.8944) -> (-360.2109, 48.8944)
  spline S563 degree 2 poles (-360.7485, 49.6357) (-360.7485, 49.548) (-360.6353, 49.432) (-360.5306, 49.432) knots 0 0 0 1 2 2 2
  spline S564 degree 2 poles (-360.5306, 49.432) (-360.3892, 49.432) (-360.2109, 49.6442) (-360.2109, 49.8111) knots 0 0 0 1 2 2 2
  line L611 (-360.2109, 49.8111) -> (-360.2109, 49.8931)
  line L612 (-360.2109, 49.8931) -> (-360.5193, 49.8507)
  spline S565 degree 2 poles (-360.5193, 49.8507) (-360.7485, 49.8111) (-360.7485, 49.6357) knots 0 0 0 1 1 1
  spline S566 degree 2 poles (-356.5187, 50.0488) (-356.5187, 49.6923) (-356.7535, 49.1405) (-357.1892, 48.8406) (-357.4637, 48.8406) knots 0 0 0 1 2 3 3 3
  spline S567 degree 2 poles (-357.4637, 48.8406) (-357.673, 48.8406) (-357.9729, 48.9962) (-358.0606, 49.1207) knots 0 0 0 1 2 2 2
  line L613 (-358.0606, 49.1207) -> (-358.0691, 49.1207)
  line L614 (-358.0691, 49.1207) -> (-358.0691, 48.8944)
  line L615 (-358.0691, 48.8944) -> (-358.9745, 48.8944)
  line L616 (-358.9745, 48.8944) -> (-358.9745, 52.1198)
  line L617 (-358.9745, 52.1198) -> (-358.0691, 52.1198)
  line L618 (-358.0691, 52.1198) -> (-358.0691, 50.7787)
  line L619 (-358.0691, 50.7787) -> (-358.0606, 50.7787)
  spline S568 degree 2 poles (-358.0606, 50.7787) (-357.9531, 50.94) (-357.591, 51.1267) (-357.3703, 51.1267) knots 0 0 0 1 2 2 2
  spline S569 degree 2 poles (-357.3703, 51.1267) (-356.96, 51.1267) (-356.5187, 50.5778) (-356.5187, 50.0488) knots 0 0 0 1 2 2 2
  spline S570 degree 2 poles (-357.4382, 50.0233) (-357.4382, 50.2411) (-357.6051, 50.4618) (-357.7636, 50.4618) knots 0 0 0 1 2 2 2
  spline S571 degree 2 poles (-357.7636, 50.4618) (-357.9022, 50.4618) (-358.0861, 50.2298) (-358.0861, 50.0459) knots 0 0 0 1 2 2 2
  line L620 (-358.0861, 50.0459) -> (-358.0861, 49.9129)
  spline S572 degree 2 poles (-358.0861, 49.9129) (-358.0861, 49.7262) (-357.9192, 49.5055) (-357.7805, 49.5055) knots 0 0 0 1 2 2 2
  spline S573 degree 2 poles (-357.7805, 49.5055) (-357.6164, 49.5055) (-357.4382, 49.7743) (-357.4382, 50.0233) knots 0 0 0 1 2 2 2
  line L621 (-356.1763, 48.8944) -> (-356.1763, 51.073)
  line L622 (-356.1763, 51.073) -> (-355.2709, 51.073)
  line L623 (-355.2709, 51.073) -> (-355.2709, 48.8944)
  line L624 (-355.2709, 48.8944) -> (-356.1763, 48.8944)
  spline S574 degree 2 poles (-355.2172, 51.6615) (-355.2172, 51.4691) (-355.4973, 51.2314) (-355.7236, 51.2314) knots 0 0 0 1 2 2 2
  spline S575 degree 2 poles (-355.7236, 51.2314) (-355.9443, 51.2314) (-356.2272, 51.4776) (-356.2272, 51.6615) knots 0 0 0 1 2 2 2
  spline S576 degree 2 poles (-356.2272, 51.6615) (-356.2272, 51.8482) (-355.9528, 52.0802) (-355.7236, 52.0802) knots 0 0 0 1 2 2 2
  spline S577 degree 2 poles (-355.7236, 52.0802) (-355.4973, 52.0802) (-355.2172, 51.8482) (-355.2172, 51.6615) knots 0 0 0 1 2 2 2
  spline S578 degree 2 poles (-352.4133, 50.0233) (-352.4133, 49.4716) (-353.0782, 48.8406) (-353.6752, 48.8406) knots 0 0 0 1 2 2 2
  spline S579 degree 2 poles (-353.6752, 48.8406) (-354.2694, 48.8406) (-354.9314, 49.4546) (-354.9314, 49.9978) knots 0 0 0 1 2 2 2
  spline S580 degree 2 poles (-354.9314, 49.9978) (-354.9314, 50.343) (-354.6202, 50.8551) (-354.0458, 51.1267) (-353.6724, 51.1267) knots 0 0 0 1 2 3 3 3
  spline S581 degree 2 poles (-353.6724, 51.1267) (-353.2848, 51.1267) (-352.7161, 50.841) (-352.4133, 50.3345) (-352.4133, 50.0233) knots 0 0 0 1 2 3 3 3
  spline S582 degree 2 poles (-353.3329, 50.0176) (-353.3329, 50.4618) (-353.6724, 50.4618) knots 0 0 0 1 1 1
  spline S583 degree 2 poles (-353.6724, 50.4618) (-354.0119, 50.4618) (-354.0119, 49.9978) knots 0 0 0 1 1 1
  spline S584 degree 2 poles (-354.0119, 49.9978) (-354.0119, 49.5055) (-353.6667, 49.5055) knots 0 0 0 1 1 1
  spline S585 degree 2 poles (-353.6667, 49.5055) (-353.3329, 49.5055) (-353.3329, 50.0176) knots 0 0 0 1 1 1
  spline S586 degree 2 poles (-398.07, 43.9961) (-398.07, 43.832) (-398.2397, 43.5406) (-398.5311, 43.3736) (-398.6924, 43.3736) knots 0 0 0 1 2 3 3 3
  spline S587 degree 2 poles (-398.6924, 43.3736) (-398.9442, 43.3736) (-399.3064, 43.7358) (-399.3064, 43.9961) knots 0 0 0 1 2 2 2
  spline S588 degree 2 poles (-399.3064, 43.9961) (-399.3064, 44.2479) (-398.9499, 44.61) (-398.6924, 44.61) knots 0 0 0 1 2 2 2
  spline S589 degree 2 poles (-398.6924, 44.61) (-398.4293, 44.61) (-398.07, 44.2422) (-398.07, 43.9961) knots 0 0 0 1 2 2 2
  line L625 (-387.4006, 42.9577) -> (-387.4006, 44.6299)
  spline S590 degree 2 poles (-387.4006, 44.6299) (-387.4006, 44.8647) (-387.3865, 45.1476) knots 0 0 0 1 1 1
  line L626 (-387.3865, 45.1476) -> (-387.378, 45.2891)
  line L627 (-387.378, 45.2891) -> (-387.4035, 45.2891)
  spline S591 degree 2 poles (-387.4035, 45.2891) (-387.4742, 44.9298) (-387.5081, 44.7911) knots 0 0 0 1 1 1
  line L628 (-387.5081, 44.7911) -> (-387.958, 42.9577)
  line L629 (-387.958, 42.9577) -> (-388.8209, 42.9577)
  line L630 (-388.8209, 42.9577) -> (-389.2906, 44.7713)
  spline S592 degree 2 poles (-389.2906, 44.7713) (-389.3104, 44.8392) (-389.3925, 45.2891) knots 0 0 0 1 1 1
  line L631 (-389.3925, 45.2891) -> (-389.4179, 45.2891)
  spline S593 degree 2 poles (-389.4179, 45.2891) (-389.3868, 44.5733) (-389.3868, 44.395) knots 0 0 0 1 1 1
  line L632 (-389.3868, 44.395) -> (-389.3868, 42.9577)
  line L633 (-389.3868, 42.9577) -> (-390.1932, 42.9577)
  line L634 (-390.1932, 42.9577) -> (-390.1932, 46.0077)
  line L635 (-390.1932, 46.0077) -> (-388.8181, 46.0077)
  line L636 (-388.8181, 46.0077) -> (-388.3994, 44.3526)
  spline S594 degree 2 poles (-388.3994, 44.3526) (-388.3824, 44.3017) (-388.3343, 43.9876) (-388.3286, 43.9027) knots 0 0 0 1 2 2 2
  line L637 (-388.3286, 43.9027) -> (-388.3145, 43.9027)
  spline S595 degree 2 poles (-388.3145, 43.9027) (-388.2919, 44.0951) (-388.2409, 44.3611) knots 0 0 0 1 1 1
  line L638 (-388.2409, 44.3611) -> (-387.8505, 46.0077)
  line L639 (-387.8505, 46.0077) -> (-386.4952, 46.0077)
  line L640 (-386.4952, 46.0077) -> (-386.4952, 42.9577)
  line L641 (-386.4952, 42.9577) -> (-387.4006, 42.9577)
  spline S596 degree 2 poles (-385.1938, 43.7895) (-385.1711, 43.6481) (-384.8939, 43.4896) (-384.6675, 43.4896) knots 0 0 0 1 2 2 2
  spline S597 degree 2 poles (-384.6675, 43.4896) (-384.3506, 43.4896) (-384.0677, 43.6113) knots 0 0 0 1 1 1
  line L642 (-384.0677, 43.6113) -> (-384.0677, 43.0369)
  spline S598 degree 2 poles (-384.0677, 43.0369) (-384.3959, 42.904) (-384.8684, 42.904) knots 0 0 0 1 1 1
  spline S599 degree 2 poles (-384.8684, 42.904) (-385.4371, 42.904) (-386.0708, 43.4868) (-386.0708, 43.9989) knots 0 0 0 1 2 2 2
  spline S600 degree 2 poles (-386.0708, 43.9989) (-386.0708, 44.3497) (-385.7936, 44.8845) (-385.2475, 45.1901) (-384.9165, 45.1901) knots 0 0 0 1 2 3 3 3
  spline S601 degree 2 poles (-384.9165, 45.1901) (-384.5798, 45.1901) (-384.0988, 44.9269) (-383.8498, 44.4488) (-383.8498, 44.1291) knots 0 0 0 1 2 3 3 3
  line L643 (-383.8498, 44.1291) -> (-383.8498, 43.7895)
  line L644 (-383.8498, 43.7895) -> (-385.1938, 43.7895)
  spline S602 degree 2 poles (-384.6505, 44.2649) (-384.6505, 44.6412) (-384.9193, 44.6412) knots 0 0 0 1 1 1
  spline S603 degree 2 poles (-384.9193, 44.6412) (-385.0325, 44.6412) (-385.1853, 44.4346) (-385.1994, 44.2649) knots 0 0 0 1 2 2 2
  line L645 (-385.1994, 44.2649) -> (-384.6505, 44.2649)
  line L646 (-382.124, 42.9577) -> (-382.124, 44.146)
  spline S604 degree 2 poles (-382.124, 44.146) (-382.124, 44.3497) (-382.2456, 44.5252) (-382.3814, 44.5252) knots 0 0 0 1 2 2 2
  spline S605 degree 2 poles (-382.3814, 44.5252) (-382.4974, 44.5252) (-382.6304, 44.3413) (-382.6304, 44.1998) knots 0 0 0 1 2 2 2
  line L647 (-382.6304, 44.1998) -> (-382.6304, 42.9577)
  line L648 (-382.6304, 42.9577) -> (-383.5358, 42.9577)
  line L649 (-383.5358, 42.9577) -> (-383.5358, 45.1363)
  line L650 (-383.5358, 45.1363) -> (-382.6304, 45.1363)
  line L651 (-382.6304, 45.1363) -> (-382.6304, 44.7968)
  line L652 (-382.6304, 44.7968) -> (-382.6219, 44.7968)
  spline S606 degree 2 poles (-382.6219, 44.7968) (-382.5144, 44.9835) (-382.1466, 45.1901) (-381.9316, 45.1901) knots 0 0 0 1 2 2 2
  spline S607 degree 2 poles (-381.9316, 45.1901) (-381.2186, 45.1901) (-381.2186, 44.2875) knots 0 0 0 1 1 1
  line L653 (-381.2186, 44.2875) -> (-381.2186, 42.9577)
  line L654 (-381.2186, 42.9577) -> (-382.124, 42.9577)
  line L655 (-380.8083, 42.9577) -> (-380.8083, 45.1363)
  line L656 (-380.8083, 45.1363) -> (-379.9029, 45.1363)
  line L657 (-379.9029, 45.1363) -> (-379.9029, 42.9577)
  line L658 (-379.9029, 42.9577) -> (-380.8083, 42.9577)
  spline S608 degree 2 poles (-379.8492, 45.7248) (-379.8492, 45.5324) (-380.1293, 45.2947) (-380.3556, 45.2947) knots 0 0 0 1 2 2 2
  spline S609 degree 2 poles (-380.3556, 45.2947) (-380.5763, 45.2947) (-380.8593, 45.5409) (-380.8593, 45.7248) knots 0 0 0 1 2 2 2
  spline S610 degree 2 poles (-380.8593, 45.7248) (-380.8593, 45.9115) (-380.5848, 46.1435) (-380.3556, 46.1435) knots 0 0 0 1 2 2 2
  spline S611 degree 2 poles (-380.3556, 46.1435) (-380.1293, 46.1435) (-379.8492, 45.9115) (-379.8492, 45.7248) knots 0 0 0 1 2 2 2
  spline S612 degree 2 poles (-377.6734, 43.02) (-377.7612, 42.969) (-378.1346, 42.904) (-378.3779, 42.904) knots 0 0 0 1 2 2 2
  spline S613 degree 2 poles (-378.3779, 42.904) (-378.7231, 42.904) (-379.2663, 43.1841) (-379.5634, 43.6849) (-379.5634, 43.9989) knots 0 0 0 1 2 3 3 3
  spline S614 degree 2 poles (-379.5634, 43.9989) (-379.5634, 44.3724) (-379.2465, 44.9071) (-378.6609, 45.1901) (-378.2733, 45.1901) knots 0 0 0 1 2 3 3 3
  spline S615 degree 2 poles (-378.2733, 45.1901) (-378.0611, 45.1901) (-377.7215, 45.1335) (-377.6734, 45.0995) knots 0 0 0 1 2 2 2
  line L659 (-377.6734, 45.0995) -> (-377.6734, 44.3922)
  spline S616 degree 2 poles (-377.6734, 44.3922) (-377.7413, 44.4459) (-377.996, 44.5252) (-378.1035, 44.5252) knots 0 0 0 1 2 2 2
  spline S617 degree 2 poles (-378.1035, 44.5252) (-378.3695, 44.5252) (-378.6439, 44.2734) (-378.6439, 44.0442) knots 0 0 0 1 2 2 2
  spline S618 degree 2 poles (-378.6439, 44.0442) (-378.6439, 43.8178) (-378.3751, 43.5689) (-378.1375, 43.5689) knots 0 0 0 1 2 2 2
  spline S619 degree 2 poles (-378.1375, 43.5689) (-377.8856, 43.5689) (-377.6734, 43.6877) knots 0 0 0 1 1 1
  line L660 (-377.6734, 43.6877) -> (-377.6734, 43.02)
  line L661 (-375.908, 42.9577) -> (-375.908, 44.1998)
  spline S620 degree 2 poles (-375.908, 44.1998) (-375.908, 44.5252) (-376.1569, 44.5252) knots 0 0 0 1 1 1
  spline S621 degree 2 poles (-376.1569, 44.5252) (-376.2786, 44.5252) (-376.4059, 44.3413) (-376.4059, 44.1941) knots 0 0 0 1 2 2 2
  line L662 (-376.4059, 44.1941) -> (-376.4059, 42.9577)
  line L663 (-376.4059, 42.9577) -> (-377.3113, 42.9577)
  line L664 (-377.3113, 42.9577) -> (-377.3113, 46.1831)
  line L665 (-377.3113, 46.1831) -> (-376.4059, 46.1831)
  line L666 (-376.4059, 46.1831) -> (-376.4059, 44.842)
  line L667 (-376.4059, 44.842) -> (-376.3974, 44.842)
  spline S622 degree 2 poles (-376.3974, 44.842) (-376.2814, 45.009) (-375.9447, 45.1901) (-375.7552, 45.1901) knots 0 0 0 1 2 2 2
  spline S623 degree 2 poles (-375.7552, 45.1901) (-375.4015, 45.1901) (-375.0309, 44.7374) (-375.0309, 44.296) knots 0 0 0 1 2 2 2
  line L668 (-375.0309, 44.296) -> (-375.0309, 42.9577)
  line L669 (-375.0309, 42.9577) -> (-375.908, 42.9577)
  spline S624 degree 2 poles (-373.8426, 43.7895) (-373.8199, 43.6481) (-373.5426, 43.4896) (-373.3163, 43.4896) knots 0 0 0 1 2 2 2
  spline S625 degree 2 poles (-373.3163, 43.4896) (-372.9994, 43.4896) (-372.7165, 43.6113) knots 0 0 0 1 1 1
  line L670 (-372.7165, 43.6113) -> (-372.7165, 43.0369)
  spline S626 degree 2 poles (-372.7165, 43.0369) (-373.0447, 42.904) (-373.5172, 42.904) knots 0 0 0 1 1 1
  spline S627 degree 2 poles (-373.5172, 42.904) (-374.0859, 42.904) (-374.7196, 43.4868) (-374.7196, 43.9989) knots 0 0 0 1 2 2 2
  spline S628 degree 2 poles (-374.7196, 43.9989) (-374.7196, 44.3497) (-374.4424, 44.8845) (-373.8963, 45.1901) (-373.5653, 45.1901) knots 0 0 0 1 2 3 3 3
  spline S629 degree 2 poles (-373.5653, 45.1901) (-373.2286, 45.1901) (-372.7476, 44.9269) (-372.4986, 44.4488) (-372.4986, 44.1291) knots 0 0 0 1 2 3 3 3
  line L671 (-372.4986, 44.1291) -> (-372.4986, 43.7895)
  line L672 (-372.4986, 43.7895) -> (-373.8426, 43.7895)
  spline S630 degree 2 poles (-373.2993, 44.2649) (-373.2993, 44.6412) (-373.5681, 44.6412) knots 0 0 0 1 1 1
  spline S631 degree 2 poles (-373.5681, 44.6412) (-373.6813, 44.6412) (-373.8341, 44.4346) (-373.8482, 44.2649) knots 0 0 0 1 2 2 2
  line L673 (-373.8482, 44.2649) -> (-373.2993, 44.2649)
  line L674 (-372.1846, 42.9577) -> (-372.1846, 46.1831)
  line L675 (-372.1846, 46.1831) -> (-371.2792, 46.1831)
  line L676 (-371.2792, 46.1831) -> (-371.2792, 42.9577)
  line L677 (-371.2792, 42.9577) -> (-372.1846, 42.9577)
  line L678 (-370.8435, 42.9577) -> (-370.8435, 46.1831)
  line L679 (-370.8435, 46.1831) -> (-369.9381, 46.1831)
  line L680 (-369.9381, 46.1831) -> (-369.9381, 42.9577)
  line L681 (-369.9381, 42.9577) -> (-370.8435, 42.9577)
  line L682 (-369.5024, 42.9577) -> (-369.5024, 45.1363)
  line L683 (-369.5024, 45.1363) -> (-368.597, 45.1363)
  line L684 (-368.597, 45.1363) -> (-368.597, 42.9577)
  line L685 (-368.597, 42.9577) -> (-369.5024, 42.9577)
  spline S632 degree 2 poles (-368.5432, 45.7248) (-368.5432, 45.5324) (-368.8234, 45.2947) (-369.0497, 45.2947) knots 0 0 0 1 2 2 2
  spline S633 degree 2 poles (-369.0497, 45.2947) (-369.2704, 45.2947) (-369.5533, 45.5409) (-369.5533, 45.7248) knots 0 0 0 1 2 2 2
  spline S634 degree 2 poles (-369.5533, 45.7248) (-369.5533, 45.9115) (-369.2789, 46.1435) (-369.0497, 46.1435) knots 0 0 0 1 2 2 2
  spline S635 degree 2 poles (-369.0497, 46.1435) (-368.8234, 46.1435) (-368.5432, 45.9115) (-368.5432, 45.7248) knots 0 0 0 1 2 2 2
  line L686 (-364.9557, 42.9577) -> (-365.0887, 43.5179)
  line L687 (-365.0887, 43.5179) -> (-365.9997, 43.5179)
  line L688 (-365.9997, 43.5179) -> (-366.144, 42.9577)
  line L689 (-366.144, 42.9577) -> (-367.1371, 42.9577)
  line L690 (-367.1371, 42.9577) -> (-366.0874, 46.0077)
  line L691 (-366.0874, 46.0077) -> (-364.9472, 46.0077)
  line L692 (-364.9472, 46.0077) -> (-363.9569, 42.9577)
  line L693 (-363.9569, 42.9577) -> (-364.9557, 42.9577)
  line L694 (-365.5329, 45.3428) -> (-365.5527, 45.3428)
  spline S636 degree 2 poles (-365.5527, 45.3428) (-365.5583, 45.2919) (-365.6093, 45.0571) (-365.8413, 44.1715) knots 0 0 0 1 2 2 2
  line L695 (-365.8413, 44.1715) -> (-365.2584, 44.1715)
  line L696 (-365.2584, 44.1715) -> (-365.4706, 45.0005)
  spline S637 degree 2 poles (-365.4706, 45.0005) (-365.5159, 45.1844) (-365.5329, 45.3428) knots 0 0 0 1 1 1
  line L697 (-363.6825, 42.9577) -> (-363.6825, 46.1831)
  line L698 (-363.6825, 46.1831) -> (-362.7771, 46.1831)
  line L699 (-362.7771, 46.1831) -> (-362.7771, 42.9577)
  line L700 (-362.7771, 42.9577) -> (-363.6825, 42.9577)
  spline S638 degree 2 poles (-359.8855, 44.1121) (-359.8855, 43.7556) (-360.1204, 43.2039) (-360.5561, 42.904) (-360.8305, 42.904) knots 0 0 0 1 2 3 3 3
  spline S639 degree 2 poles (-360.8305, 42.904) (-361.0399, 42.904) (-361.3398, 43.0596) (-361.4275, 43.1841) knots 0 0 0 1 2 2 2
  line L701 (-361.4275, 43.1841) -> (-361.436, 43.1841)
  line L702 (-361.436, 43.1841) -> (-361.436, 42.9577)
  line L703 (-361.436, 42.9577) -> (-362.3414, 42.9577)
  line L704 (-362.3414, 42.9577) -> (-362.3414, 46.1831)
  line L705 (-362.3414, 46.1831) -> (-361.436, 46.1831)
  line L706 (-361.436, 46.1831) -> (-361.436, 44.842)
  line L707 (-361.436, 44.842) -> (-361.4275, 44.842)
  spline S640 degree 2 poles (-361.4275, 44.842) (-361.32, 45.0033) (-360.9579, 45.1901) (-360.7372, 45.1901) knots 0 0 0 1 2 2 2
  spline S641 degree 2 poles (-360.7372, 45.1901) (-360.3269, 45.1901) (-359.8855, 44.6412) (-359.8855, 44.1121) knots 0 0 0 1 2 2 2
  spline S642 degree 2 poles (-360.8051, 44.0866) (-360.8051, 44.3045) (-360.972, 44.5252) (-361.1304, 44.5252) knots 0 0 0 1 2 2 2
  spline S643 degree 2 poles (-361.1304, 44.5252) (-361.2691, 44.5252) (-361.453, 44.2932) (-361.453, 44.1093) knots 0 0 0 1 2 2 2
  line L708 (-361.453, 44.1093) -> (-361.453, 43.9763)
  spline S644 degree 2 poles (-361.453, 43.9763) (-361.453, 43.7895) (-361.2861, 43.5689) (-361.1474, 43.5689) knots 0 0 0 1 2 2 2
  spline S645 degree 2 poles (-361.1474, 43.5689) (-360.9833, 43.5689) (-360.8051, 43.8376) (-360.8051, 44.0866) knots 0 0 0 1 2 2 2
  spline S646 degree 2 poles (-358.7623, 43.7895) (-358.7397, 43.6481) (-358.4624, 43.4896) (-358.2361, 43.4896) knots 0 0 0 1 2 2 2
  spline S647 degree 2 poles (-358.2361, 43.4896) (-357.9192, 43.4896) (-357.6362, 43.6113) knots 0 0 0 1 1 1
  line L709 (-357.6362, 43.6113) -> (-357.6362, 43.0369)
  spline S648 degree 2 poles (-357.6362, 43.0369) (-357.9644, 42.904) (-358.4369, 42.904) knots 0 0 0 1 1 1
  spline S649 degree 2 poles (-358.4369, 42.904) (-359.0056, 42.904) (-359.6394, 43.4868) (-359.6394, 43.9989) knots 0 0 0 1 2 2 2
  spline S650 degree 2 poles (-359.6394, 43.9989) (-359.6394, 44.3497) (-359.3621, 44.8845) (-358.8161, 45.1901) (-358.485, 45.1901) knots 0 0 0 1 2 3 3 3
  spline S651 degree 2 poles (-358.485, 45.1901) (-358.1484, 45.1901) (-357.6674, 44.9269) (-357.4184, 44.4488) (-357.4184, 44.1291) knots 0 0 0 1 2 3 3 3
  line L710 (-357.4184, 44.1291) -> (-357.4184, 43.7895)
  line L711 (-357.4184, 43.7895) -> (-358.7623, 43.7895)
  spline S652 degree 2 poles (-358.2191, 44.2649) (-358.2191, 44.6412) (-358.4879, 44.6412) knots 0 0 0 1 1 1
  spline S653 degree 2 poles (-358.4879, 44.6412) (-358.601, 44.6412) (-358.7538, 44.4346) (-358.768, 44.2649) knots 0 0 0 1 2 2 2
  line L712 (-358.768, 44.2649) -> (-358.2191, 44.2649)
  spline S654 degree 2 poles (-355.4662, 44.3611) (-355.5171, 44.3837) (-355.6925, 44.4205) (-355.7491, 44.4205) knots 0 0 0 1 2 2 2
  spline S655 degree 2 poles (-355.7491, 44.4205) (-356.199, 44.4205) (-356.199, 43.9027) knots 0 0 0 1 1 1
  line L713 (-356.199, 43.9027) -> (-356.199, 42.9577)
  line L714 (-356.199, 42.9577) -> (-357.1043, 42.9577)
  line L715 (-357.1043, 42.9577) -> (-357.1043, 45.1363)
  line L716 (-357.1043, 45.1363) -> (-356.199, 45.1363)
  line L717 (-356.199, 45.1363) -> (-356.199, 44.7543)
  line L718 (-356.199, 44.7543) -> (-356.1905, 44.7543)
  spline S656 degree 2 poles (-356.1905, 44.7543) (-356.1084, 44.9609) (-355.8, 45.1759) (-355.5963, 45.1759) knots 0 0 0 1 2 2 2
  spline S657 degree 2 poles (-355.5963, 45.1759) (-355.5227, 45.1759) (-355.4662, 45.1504) knots 0 0 0 1 1 1
  line L719 (-355.4662, 45.1504) -> (-355.4662, 44.3611)
  spline S658 degree 2 poles (-353.6724, 42.986) (-353.7346, 42.9577) (-354.0147, 42.904) (-354.2128, 42.904) knots 0 0 0 1 2 2 2
  spline S659 degree 2 poles (-354.2128, 42.904) (-354.5919, 42.904) (-355.0191, 43.3199) (-355.0191, 43.7075) knots 0 0 0 1 2 2 2
  line L720 (-355.0191, 43.7075) -> (-355.0191, 44.5082)
  line L721 (-355.0191, 44.5082) -> (-355.3615, 44.5082)
  line L722 (-355.3615, 44.5082) -> (-355.3615, 45.1363)
  line L723 (-355.3615, 45.1363) -> (-355.0191, 45.1363)
  line L724 (-355.0191, 45.1363) -> (-355.0191, 45.5635)
  line L725 (-355.0191, 45.5635) -> (-354.1251, 45.8097)
  line L726 (-354.1251, 45.8097) -> (-354.1251, 45.1363)
  line L727 (-354.1251, 45.1363) -> (-353.6724, 45.1363)
  line L728 (-353.6724, 45.1363) -> (-353.6724, 44.5082)
  line L729 (-353.6724, 44.5082) -> (-354.1251, 44.5082)
  line L730 (-354.1251, 44.5082) -> (-354.1251, 43.8546)
  spline S660 degree 2 poles (-354.1251, 43.8546) (-354.1251, 43.5689) (-353.8987, 43.5689) knots 0 0 0 1 1 1
  spline S661 degree 2 poles (-353.8987, 43.5689) (-353.7912, 43.5689) (-353.6724, 43.6141) knots 0 0 0 1 1 1
  line L731 (-353.6724, 43.6141) -> (-353.6724, 42.986)
  spline S662 degree 2 poles (-350.9676, 44.0866) (-350.9676, 43.5349) (-351.6324, 42.904) (-352.2294, 42.904) knots 0 0 0 1 2 2 2
  spline S663 degree 2 poles (-352.2294, 42.904) (-352.8236, 42.904) (-353.4856, 43.5179) (-353.4856, 44.0612) knots 0 0 0 1 2 2 2
  spline S664 degree 2 poles (-353.4856, 44.0612) (-353.4856, 44.4063) (-353.1744, 44.9184) (-352.6001, 45.1901) (-352.2266, 45.1901) knots 0 0 0 1 2 3 3 3
  spline S665 degree 2 poles (-352.2266, 45.1901) (-351.839, 45.1901) (-351.2703, 44.9043) (-350.9676, 44.3978) (-350.9676, 44.0866) knots 0 0 0 1 2 3 3 3
  spline S666 degree 2 poles (-351.8871, 44.081) (-351.8871, 44.5252) (-352.2266, 44.5252) knots 0 0 0 1 1 1
  spline S667 degree 2 poles (-352.2266, 44.5252) (-352.5661, 44.5252) (-352.5661, 44.0612) knots 0 0 0 1 1 1
  spline S668 degree 2 poles (-352.5661, 44.0612) (-352.5661, 43.5689) (-352.2209, 43.5689) knots 0 0 0 1 1 1
  spline S669 degree 2 poles (-352.2209, 43.5689) (-351.8871, 43.5689) (-351.8871, 44.081) knots 0 0 0 1 1 1
  spline S670 degree 2 poles (-398.07, 38.0594) (-398.07, 37.8953) (-398.2397, 37.6039) (-398.5311, 37.437) (-398.6924, 37.437) knots 0 0 0 1 2 3 3 3
  spline S671 degree 2 poles (-398.6924, 37.437) (-398.9442, 37.437) (-399.3064, 37.7991) (-399.3064, 38.0594) knots 0 0 0 1 2 2 2
  spline S672 degree 2 poles (-399.3064, 38.0594) (-399.3064, 38.3112) (-398.9499, 38.6734) (-398.6924, 38.6734) knots 0 0 0 1 2 2 2
  spline S673 degree 2 poles (-398.6924, 38.6734) (-398.4293, 38.6734) (-398.07, 38.3056) (-398.07, 38.0594) knots 0 0 0 1 2 2 2
  line L732 (-389.2736, 39.3524) -> (-389.2736, 38.8035)
  line L733 (-389.2736, 38.8035) -> (-388.3682, 38.8035)
  line L734 (-388.3682, 38.8035) -> (-388.3682, 38.0849)
  line L735 (-388.3682, 38.0849) -> (-389.2736, 38.0849)
  line L736 (-389.2736, 38.0849) -> (-389.2736, 37.0211)
  line L737 (-389.2736, 37.0211) -> (-390.1932, 37.0211)
  line L738 (-390.1932, 37.0211) -> (-390.1932, 40.0711)
  line L739 (-390.1932, 40.0711) -> (-388.2805, 40.0711)
  line L740 (-388.2805, 40.0711) -> (-388.2805, 39.3524)
  line L741 (-388.2805, 39.3524) -> (-389.2736, 39.3524)
  spline S674 degree 2 poles (-387.1375, 37.8529) (-387.1149, 37.7114) (-386.8376, 37.553) (-386.6112, 37.553) knots 0 0 0 1 2 2 2
  spline S675 degree 2 poles (-386.6112, 37.553) (-386.2944, 37.553) (-386.0114, 37.6746) knots 0 0 0 1 1 1
  line L742 (-386.0114, 37.6746) -> (-386.0114, 37.1003)
  spline S676 degree 2 poles (-386.0114, 37.1003) (-386.3396, 36.9673) (-386.8121, 36.9673) knots 0 0 0 1 1 1
  spline S677 degree 2 poles (-386.8121, 36.9673) (-387.3808, 36.9673) (-388.0146, 37.5501) (-388.0146, 38.0622) knots 0 0 0 1 2 2 2
  spline S678 degree 2 poles (-388.0146, 38.0622) (-388.0146, 38.4131) (-387.7373, 38.9478) (-387.1913, 39.2534) (-386.8602, 39.2534) knots 0 0 0 1 2 3 3 3
  spline S679 degree 2 poles (-386.8602, 39.2534) (-386.5235, 39.2534) (-386.0426, 38.9903) (-385.7936, 38.5121) (-385.7936, 38.1924) knots 0 0 0 1 2 3 3 3
  line L743 (-385.7936, 38.1924) -> (-385.7936, 37.8529)
  line L744 (-385.7936, 37.8529) -> (-387.1375, 37.8529)
  spline S680 degree 2 poles (-386.5943, 38.3282) (-386.5943, 38.7045) (-386.8631, 38.7045) knots 0 0 0 1 1 1
  spline S681 degree 2 poles (-386.8631, 38.7045) (-386.9762, 38.7045) (-387.129, 38.498) (-387.1432, 38.3282) knots 0 0 0 1 2 2 2